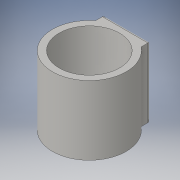
# Autodesk Inventor part: ROV Motor couppling
Saved by Autodesk Inventor 2016 (Build 200138000, 138)
## iProperties
Created: 2017-03-07
Part Number: ROV Motor couppling
Material: Generic
Document SubType Name: Modeling
Designer: Student
Density: 1 g/cm^3
Appearance: Default
Author: Student
Autodesk Inventor part; units mm, degrees
ref_plane "YZ Plane" through (0, 0, 0) normal (1, 0, 0) x (0, 1, 0)
ref_plane "XZ Plane" through (0, 0, 0) normal (0, 1, 0) x (-1, 0, 0)
ref_plane "XY Plane" through (0, 0, 0) normal (0, 0, 1) x (1, 0, 0)
sketch "Sketch1" plane through (0, 0, 0) normal (0, 1, 0) x (-1, 0, 0)
  circle A0 centre (0, 0) radius 16.7005
  circle A1 centre (0, 0) radius 20.32
  dimension "d1" = 33.401
  dimension "d2" = 40.64
  constraints: 2 centre point, 1 coincident
  measures "d1" diameter of A0
  measures "d2" diameter of A1
extrude "Extrusion1" add sketch "Sketch1" along normal blind 38.1
sketch "Sketch2" plane through (0, 38.1, 0) normal (0, 1, 0) x (1, 0, 0)
  line L0 (0, 0) -> (0, 17.78) construction
  line L1 (0, 17.78) -> (-12.5588, 15.9743)
  circle A0 centre (0, 0) radius 20.32 projected
  line L2 (0, 17.78) -> (12.5588, 15.9743)
  line L3 (-12.5588, 15.9743) -> (-12.5588, 21.0543)
  line L4 (-12.5588, 21.0543) -> (0, 21.0543)
  line L5 (12.5588, 15.9743) -> (12.5588, 21.0543)
  line L6 (12.5588, 21.0543) -> (0, 21.0543)
  dimension "d5" = 17.78
  dimension "d6" = 5.08
  constraints: 14 end point, 2 symmetric about line, 2 vertical, 1 perpendicular, 2 other
  measures "d5" distance of L0.start L0.end
  measures "d6" distance of L1.end L3.end
extrude "Extrusion2" add sketch "Sketch2" against normal blind 38.1 contours L1 A0 L2 | L3 L4 L6 L5 A0 picked at (-7.0969, 17.3675)
sketch "Sketch3" plane through (12.5588, 38.1, -21.0543) normal (0, 0, -1) x (-1, 0, 0)
  circle A0 centre (21.5758, -19.05) radius 1.2319
  line L0 (25.1176, -38.1) -> (0, -38.1) projected
  line L1 (25.1176, 0) -> (25.1176, -38.1) projected
  line L2 (12.5588, -38.1) -> (12.5588, 17.1945) construction
  circle A1 centre (3.5418, -19.05) radius 1.2319
  circle A2 centre (12.5588, -27.9654) radius 1.2319
  circle A3 centre (12.5588, -10.1346) radius 1.2319
  line L3 (25.1176, 0) -> (0, 0) projected
  dimension "d9" = 2.4638
  dimension "d10" = 19.05
  dimension "d12" = 18.034
  dimension "d13" = 2.4638
  dimension "d14" = 2.4638
  dimension "d16" = 10.1346
  dimension "d17" = 10.1346
  constraints: 4 centre point, 2 end point, 2 point on line, 1 symmetric about line, 1 vertical, 1 other
  measures "d9" diameter of A0
  measures "d10" distance from line of L0 A0.centre
  measures "d12" distance of A1.centre A0.centre
  measures "d13" diameter of A2
  measures "d14" diameter of A3
  measures "d16" distance from line of L0 A2.centre
  measures "d17" distance from line of L3 A3.centre
extrude "Extrusion3" cut sketch "Sketch3" against normal blind 2.54
fillet "Fillet1" radius 1.27 4 edges at (0, 0, -21.0543) (-12.5588, 19.05, -21.0543) (12.5588, 19.05, -21.0543) (0, 38.1, -21.0543)
body "Solid1"
